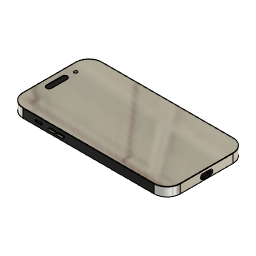
Smartphone_ (Autodesk Fusion 360 design; units mm, degrees)
Autodesk Fusion 360 part; units mm, degrees
sketch "Skizze1" plane through (0, 0, 0) normal (0, 0, 1) x (1, 0, 0)
  line L0 (0, 0) -> (150.9, 0)
  line L1 (150.9, 0) -> (150.9, 75.7)
  line L2 (150.9, 75.7) -> (0, 75.7)
  line L3 (0, 75.7) -> (0, 0)
  dimension "d1" = 150.9
  dimension "d2" = 75.7
  constraint horizontal L0
  constraint vertical L1
  constraint horizontal L2
  constraint vertical L3
  constraint coincident L0.start L3.end
  measures "d1" distance of L0.start L0.end
  measures "d2" distance of L0.start L2.end
extrude "Extrusion1" add sketch "Skizze1" along normal blind 8.3 makes body 1
fillet "Abrundung1" radius 12.5 4 edges at (150.9, 0, 4.15) (0, 0, 4.15) (150.9, 75.7, 4.15) (0, 75.7, 4.15) on bodies 1
sketch "Skizze2" plane through (0, 0, 8.3) normal (0, 0, 1) x (-1, 0, 0)
  arc A0 (-12.5, -75.7) -> (0, -63.2) centre (-12.5, -63.2) ccw
  line L0 (0, -63.2) -> (0, -12.5)
  arc A1 (0, -12.5) -> (-12.5, 0) centre (-12.5, -12.5) ccw
  line L1 (-12.5, 0) -> (-138.4, 0)
  arc A2 (-138.4, 0) -> (-150.9, -12.5) centre (-138.4, -12.5) ccw
  line L2 (-150.9, -12.5) -> (-150.9, -63.2)
  arc A3 (-150.9, -63.2) -> (-138.4, -75.7) centre (-138.4, -63.2) ccw
  line L3 (-138.4, -75.7) -> (-12.5, -75.7)
  line L4 (-5, -30) -> (-5, -45)
  line L5 (-10, -30) -> (-10, -45)
  arc A4 (-10, -45) -> (-5, -45) centre (-7.5, -45) ccw
  arc A5 (-5, -30) -> (-10, -30) centre (-7.5, -30) ccw
  constraint vertical L4
  constraint vertical L5
  constraint tangent L5 A4
  constraint tangent L4 A4
  constraint tangent L4 A5
  constraint tangent L5 A5
sketch "Skizze3" plane through (150.9, 0, 0) normal (1, 0, 0) x (0, 1, 0)
  line L0 (63.2, 0) -> (63.2, 8.3)
  line L1 (63.2, 8.3) -> (12.5, 8.3)
  line L2 (12.5, 8.3) -> (12.5, 0)
  line L3 (12.5, 0) -> (63.2, 0)
  line L4 (34.5, 5) -> (41.2, 5)
  arc A0 (41.2, 2) -> (41.2, 5) centre (41.2, 3.5) ccw
  line L5 (41.2, 2) -> (34.5, 2)
  arc A1 (34.5, 5) -> (34.5, 2) centre (34.5, 3.5) ccw
  dimension "d9" = 22
  dimension "d11" = 22
  constraint parallel L3 L4
  constraint tangent L4 A0
  constraint tangent A0 L5
  constraint parallel L4 L5
  constraint tangent L5 A1
  constraint tangent L4 A1
  measures "d9" distance of L2 A1.centre
  measures "d11" distance of L0 A0.centre
extrude "Extrusion2" cut sketch "Skizze3" against normal blind 4 contours L4 A0 L5 A1 bodies 1
chamfer "Fase1" distance 1 angle 45 4 edges at (150.9, 37.85, 5) (150.9, 42.7, 3.5) (150.9, 37.85, 2) (150.9, 33, 3.5) on bodies 1
extrude "Extrusion3" add sketch "Skizze2" along normal blind 0.5 separate body makes body 2
sketch "Skizze4" plane through (0, 75.7, 0) normal (0, 1, 0) x (-1, 0, 0)
  line L0 (-12.5, 0) -> (-12.5, 8.3)
  line L1 (-12.5, 8.3) -> (-138.4, 8.3)
  line L2 (-138.4, 8.3) -> (-138.4, 0)
  line L3 (-138.4, 0) -> (-12.5, 0)
  line L4 (-41.1644, 5.2368) -> (-38.1644, 5.2368)
  line L5 (-41.1644, 3.2368) -> (-38.1644, 3.2368)
  arc A0 (-38.1644, 3.2368) -> (-38.1644, 5.2368) centre (-38.1644, 4.2368) ccw
  line L6 (-41.1644, 5.2368) -> (-47.1644, 5.2368)
  arc A1 (-47.1644, 5.2368) -> (-47.1644, 3.2368) centre (-47.1644, 4.2368) ccw
  line L7 (-47.1644, 3.2368) -> (-41.1644, 3.2368)
  constraint parallel L1 L4
  constraint horizontal L5
  constraint tangent L5 A0
  constraint tangent L4 A0
  constraint parallel L4 L6
  constraint tangent L6 A1
  constraint tangent A1 L7
extrude "Extrusion4" add sketch "Skizze4" along normal blind 1 contours L4 L5 A0 L6 A1 L7 bodies 1
sketch "Skizze5" plane through (0, 0, 0) normal (0, -1, 0) x (1, 0, 0)
  line L0 (12.5, 8.3) -> (12.5, 0)
  line L1 (12.5, 0) -> (138.4, 0)
  line L2 (138.4, 0) -> (138.4, 8.3)
  line L3 (138.4, 8.3) -> (12.5, 8.3)
  line L4 (25, 5) -> (30, 5)
  arc A0 (30, 3) -> (30, 5) centre (30, 4) ccw
  line L5 (30, 3) -> (25, 3)
  arc A1 (25, 5) -> (25, 3) centre (25, 4) ccw
  line L6 (51.9078, 3.0658) -> (46.9078, 3.0658)
  line L7 (46.9078, 5.0658) -> (51.9078, 5.0658)
  arc A2 (51.9078, 3.0658) -> (51.9078, 5.0658) centre (51.9078, 4.0658) ccw
  arc A3 (46.9078, 5.0658) -> (46.9078, 3.0658) centre (46.9078, 4.0658) ccw
  line L8 (60.0657, 3.0658) -> (55.0657, 3.0658)
  line L9 (55.0657, 5.0658) -> (60.0657, 5.0658)
  arc A4 (60.0657, 3.0658) -> (60.0657, 5.0658) centre (60.0657, 4.0658) ccw
  arc A5 (55.0657, 5.0658) -> (55.0657, 3.0658) centre (55.0657, 4.0658) ccw
  constraint parallel L1 L4
  constraint tangent L4 A0
  constraint tangent A0 L5
  constraint parallel L4 L5
  constraint tangent L4 A1
  constraint tangent L5 A1
  constraint tangent L7 A2
  constraint tangent L6 A2
  constraint parallel L6 L7
  constraint tangent L7 A3
  constraint tangent L6 A3
  constraint tangent L9 A4
  constraint tangent L8 A4
  constraint parallel L8 L9
  constraint tangent L9 A5
  constraint tangent L8 A5
extrude "Extrusion5" add sketch "Skizze5" along normal blind 1 separate body contours L6 L7 A2 A3 | L8 L9 A4 A5 makes body 3 at (50.2412, 0, 3.7325) makes body 4 at (58.399, 0, 3.7325)
move_body "Verschieben1" bodies 4 3 to x (1, 0, 0) y (0, 1, 0) z (0, 0, 1) at (-8.4551, -0.0538, -0.0538)
extrude "Extrusion6" cut sketch "Skizze5" against normal blind 0.5 contours L4 A0 L5 A1 bodies 1
sketch "Skizze6" plane through (0, 0, 8.3) normal (0, 0, 1) x (-1, 0, 0)
  arc A0 (-12.5, -75.7) -> (0, -63.2) centre (-12.5, -63.2) ccw
  line L0 (0, -63.2) -> (0, -12.5)
  arc A1 (0, -12.5) -> (-12.5, 0) centre (-12.5, -12.5) ccw
  line L1 (-12.5, 0) -> (-138.4, 0)
  arc A2 (-138.4, 0) -> (-150.9, -12.5) centre (-138.4, -12.5) ccw
  line L2 (-150.9, -12.5) -> (-150.9, -63.2)
  arc A3 (-150.9, -63.2) -> (-138.4, -75.7) centre (-138.4, -63.2) ccw
  line L3 (-138.4, -75.7) -> (-12.5, -75.7)
  circle A4 centre (-8, -55) radius 1.4142
extrude "Extrusion7" add sketch "Skizze6" along normal blind 0.5 separate body contours A4 makes body 5
move_body "Verschieben4" [rolled back]
sketch "Skizze7" plane through (0, 0, 0) normal (1, 0, 0) x (0, 1, 0)
move_body "Verschieben3" [suppressed]
move_body "Verschieben2" [suppressed]
copy_body "Körper->Berechn1" [suppressed] in component "Component"
copy_body "Körper->Berechn2" [suppressed] in component "Component'"
copy_body "Körper->Berechn3" [suppressed] in component "Component''"
copy_body "Körper->Berechn4" [suppressed] in component "Component'''"
copy_body "Körper->Berechn5" [suppressed] in component "Component''''"
